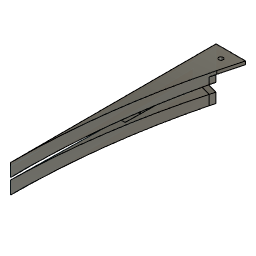
RampaZaKosuRavan v2 (Autodesk Fusion 360 design; units mm, degrees)
Autodesk Fusion 360 part; units mm, degrees
note: some values were not read from the file. Chosen so that the rebuilt part matches the saved one: which pieces of a blend or face edit are solid.
sketch "Sketch1" plane through (0, 0, 0) normal (0, 0, 1) x (1, 0, 0)
  line L0 (50, 20) -> (133, 20)
  line L1 (127.39759, 40.238898) -> (133, 20)
  line L2 (50, 20) -> (30, 20)
  line L3 (30, 20) -> (127.39759, 40.238898)
  dimension "d1" = 83
  dimension "d2" = 80
  dimension "d3" = 21
  constraint horizontal L0
  constraint parallel L0 L2
  measures "d1" distance of L0.start L0.end
extrude "Extrude1" add sketch "Sketch1" along normal blind 23 makes body 1
extrude "Extrude2" add 1 faces at (131.13253, 26.746299, 7.666667) along direction (0.96375706, 0.26678141, 0) blind 30 on bodies 1 bodies 1
sketch "Sketch2" plane through (157.589043, 43.622847, 0) normal (0.963757, 0.266781, 0) x (-0.266781, 0.963757, 0)
  line L0 (-16.206786, 0) -> (4.793214, 0)
  line L1 (4.793214, 0) -> (4.793214, 23)
  line L2 (4.793214, 23) -> (-16.206786, 23)
  line L3 (-16.206786, 23) -> (-16.206786, 0)
  line L4 (-16.206786, 23) -> (-16.206786, 20)
  line L5 (-16.206786, 20) -> (4.793214, 20)
  dimension "d8" = 3
  constraint perpendicular L2 L4
  constraint perpendicular L1 L5
extrude "Extrude3" cut sketch "Sketch2" against normal blind 30 contours L0 L1 L3 L5 picked at (-2.206786, 6.666667) bodies 1
sketch "Sketch3" plane through (0, 0, 23) normal (0, 0, 1) x (-1, 0, 0)
  line L0 (-30, -20) -> (-133, -20)
  line L1 (-133, -20) -> (-161.912712, -28.003442)
  line L2 (-161.912712, -28.003442) -> (-156.310302, -48.242341)
  line L3 (-156.310302, -48.242341) -> (-127.39759, -40.238898)
  line L4 (-127.39759, -40.238898) -> (-30, -20)
  line L5 (-156.310302, -48.242341) -> (-159.111507, -38.122892)
  line L6 (-159.111507, -38.122892) -> (-149.473936, -35.455077)
  circle A0 centre (-149.473936, -35.455077) radius 2
  dimension "d11" = 10.5
  dimension "d12" = 10
  dimension "d13" = 4
  constraint perpendicular L1 L5
  constraint perpendicular L2 L6
  measures "d13" diameter of A0
extrude "Extrude4" cut sketch "Sketch3" against normal blind 50 contours A0 picked at (-150.166062, -35.037269) bodies 1
sketch "Sketch4" plane through (0, 20, 0) normal (0, -1, 0) x (1, 0, 0)
  line L0 (30, 0) -> (133, 0)
  line L1 (133, 0) -> (133, 20)
  line L2 (133, 20) -> (133, 23)
  line L3 (133, 23) -> (30, 23)
  line L4 (30, 23) -> (30, 0)
  line L5 (133, 20) -> (133, 0)
  line L6 (133, 20) -> (133, 10)
  line L7 (133, 10) -> (30, 10)
  line L8 (30, 10) -> (30, 15)
  line L9 (30, 10) -> (30, 5)
  line L10 (30, 5) -> (133, 5)
  line L11 (133, 5) -> (30, 15)
  line L12 (30, 15) -> (133, 15)
  dimension "d16" = 10
  dimension "d17" = 5
  dimension "d18" = 5
  constraint coincident L1.end L2.start
  constraint coincident L0.end L1.start
  constraint perpendicular L0 L6
  constraint coincident L4 L7.end
  constraint perpendicular L4 L7
  constraint perpendicular L7 L8
  constraint perpendicular L7 L9
  constraint coincident L5 L10.end
  constraint perpendicular L5 L10
  constraint midpoint L6 L12.end
  measures "d16" distance of L1.end L6.end
  measures "d17" distance of L7.end L8.end
  measures "d18" distance of L7.end L9.end
extrude "Extrude5" cut sketch "Sketch4" against normal blind 8 contours L4 L7 L9 L10 L11 | L1 L5 L7 L11 | L4 L7 L8 L11 | L1 L5 L6 L7 L11 L12 picked at (81.5, 6.666667) picked at (115.833333, 8.333333) picked at (47.166667, 11.666667) picked at (81.5, 13.333333) bodies 1
sketch "Sketch5" plane through (0, 0, 0) normal (0, 0, -1) x (1, 0, 0)
  line L0 (127.39759, -40.238898) -> (133, -20)
  line L1 (133, -20) -> (30, -20)
  line L2 (30, -20) -> (127.39759, -40.238898)
  line L3 (30, -20) -> (0.627444, -13.89648)
  line L4 (0.627444, -13.89648) -> (81.5, -20)
  dimension "d21" = 30
  constraint coincident L1.end L2.start
  constraint parallel L2 L3
  constraint midpoint L1 L4.end
extrude "Extrude6" add sketch "Sketch5" against normal blind 2 contours L1 L3 L4 picked at (37.375815, -17.965493) bodies 1
extrude "Extrude7" add 1 faces at (37.375815, 17.965493, 2) along direction (0, 0, 1) blind 1 on bodies 1 bodies 1
sketch "Sketch6" plane through (0, 0, 23) normal (0, 0, 1) x (-1, 0, 0)
  circle A0 centre (-149.473936, -35.455077) radius 2
  line L0 (-30, -20) -> (-133, -20)
  line L1 (-133, -20) -> (-161.912712, -28.003442)
  line L2 (-161.912712, -28.003442) -> (-156.310302, -48.242341)
  line L3 (-156.310302, -48.242341) -> (-127.39759, -40.238898)
  line L4 (-127.39759, -40.238898) -> (-30, -20)
  line L5 (-30, -20) -> (-0.627444, -13.89648)
  line L6 (-0.627444, -13.89648) -> (-81.5, -20)
  dimension "d26" = 30
  constraint coincident L0.start L4.end
  constraint parallel L4 L5
  constraint midpoint L0 L6.end
extrude "Extrude8" add sketch "Sketch6" against normal blind 6 contours L0 L5 L6 picked at (-37.375815, -17.965493) bodies 1
sketch "Sketch7" plane through (0, 0, 0) normal (0, 0, -1) x (1, 0, 0)
  line L0 (127.39759, -40.238898) -> (133, -20)
  line L1 (133, -20) -> (81.5, -20)
  line L2 (81.5, -20) -> (0.627444, -13.89648)
  line L3 (0.627444, -13.89648) -> (127.39759, -40.238898)
  line L4 (0.627444, -13.89648) -> (-14.058834, -10.84472)
  line L5 (-14.058834, -10.84472) -> (41.063722, -16.94824)
  dimension "d30" = 15
  constraint parallel L3 L4
extrude "Extrude9" add sketch "Sketch7" against normal blind 2 contours L2 L4 L5 picked at (9.210777, -13.89648) bodies 1
sketch "Sketch8" plane through (0, 0, 23) normal (0, 0, 1) x (-1, 0, 0)
  circle A0 centre (-149.473936, -35.455077) radius 2
  line L0 (-81.5, -20) -> (-133, -20)
  line L1 (-133, -20) -> (-161.912712, -28.003442)
  line L2 (-161.912712, -28.003442) -> (-156.310302, -48.242341)
  line L3 (-156.310302, -48.242341) -> (-127.39759, -40.238898)
  line L4 (-127.39759, -40.238898) -> (-0.627444, -13.89648)
  line L5 (-0.627444, -13.89648) -> (-81.5, -20)
  line L6 (-0.627444, -13.89648) -> (14.058834, -10.84472)
  line L7 (-41.063722, -16.94824) -> (14.058834, -10.84472)
  dimension "d33" = 15
  constraint parallel L4 L6
extrude "Extrude10" add sketch "Sketch8" against normal blind 2 contours L5 L6 L7 picked at (-9.210777, -13.89648) bodies 1
sketch "Sketch9" plane through (0, 0, 0) normal (0, 0, 1) x (1, 0, 0)
  line L0 (0, 0) -> (27.195232, 0)
  line L1 (21.703887, -21) -> (0, -21)
  line L2 (0, -21) -> (0, 0)
  line L3 (0, -21) -> (0, -189.790785)
  line L4 (21.703887, -21) -> (27.195232, 0)
  line L5 (50, -50) -> (50, -133)
  line L6 (50, -50) -> (70.238898, -127.39759)
  line L7 (70.238898, -127.39759) -> (50, -133)
  line L8 (21.703887, -21) -> (0, -104) construction
  line L9 (20.238898, -26.60241) -> (0, -21) construction
  arc A0 (21.703887, -21) -> (0, -189.790785) centre (667.193566, -189.790785) ccw
  dimension "d37" = 83
  dimension "d38" = 80
  dimension "d39" = 21
  dimension "d40" = 83
  dimension "d41" = 21
  dimension "d42" = 80
  dimension "d43" = 21
  constraint coincident L0.start L2.end
  constraint horizontal L0
  constraint perpendicular L0 L2
  constraint perpendicular L1 L3
  constraint vertical L3
  constraint vertical L5
  constraint coincident L3 L8.end
  constraint collinear L4 L8
  constraint tangent L8 A0
  constraint tangent L3 A0
  measures "d37" distance of L5.start L5.end
  measures "d40" distance of L1 L8.end
  measures "d41" distance of L0 L1
extrude "Extrude11" add sketch "Sketch9" along normal blind 23 separate body contours L0 L1 L2 L4 | L1 L3 A0 picked at (16.299706, -7) picked at (10.45978, -39.525925) makes body 2
sketch "Sketch10" plane through (0, 0, 0) normal (-1, 0, 0) x (0, -1, 0)
  line L0 (0, 0) -> (189.790785, 0)
  line L1 (189.790785, 0) -> (189.790785, 23)
  line L2 (189.790785, 23) -> (0, 23)
  line L3 (0, 23) -> (0, 0)
  line L4 (189.790785, 0) -> (189.790785, 3)
  line L5 (189.790785, 3) -> (189.790785, 12)
  line L6 (189.790785, 12) -> (189.790785, 14)
  line L7 (189.790785, 14) -> (189.790785, 23)
  line L8 (0, 0) -> (21, 0)
  line L9 (21, 0) -> (21, 3)
  line L10 (21, 3) -> (21, 9)
  line L11 (21, 9) -> (21, 17)
  line L12 (21, 17) -> (21, 23)
  line L13 (21, 17) -> (189.790785, 14)
  line L14 (21, 9) -> (189.790785, 12)
  dimension "d46" = 3
  dimension "d47" = 9
  dimension "d48" = 2
  dimension "d49" = 21
  dimension "d50" = 3
  dimension "d51" = 6
  dimension "d52" = 8
  constraint perpendicular L0 L4
  constraint parallel L1 L5
  constraint parallel L1 L6
  constraint coincident L0.start L3.end
  constraint perpendicular L3 L8
  constraint perpendicular L8 L9
  constraint parallel L9 L10
  constraint parallel L10 L11
  constraint coincident L2 L12.end
  constraint perpendicular L2 L12
  measures "d49" distance of L0.start L8.end
  measures "d50" distance of L8.end L9.end
  measures "d51" distance of L9.end L10.end
  measures "d52" distance of L10.end L11.end
extrude "Extrude12" cut sketch "Sketch10" against normal blind 50 contours L1 L6 L11 L13 L14 picked at (77.263595, 13.333333) bodies 2
sketch "Sketch11" plane through (0, 0, 0) normal (-1, 0, 0) x (0, -1, 0)
  line L0 (21, 17) -> (189.790785, 14)
  line L1 (189.790785, 14) -> (189.790785, 23)
  line L2 (189.790785, 23) -> (0, 23)
  line L3 (0, 23) -> (0, 0)
  line L4 (0, 0) -> (189.790785, 0)
  line L5 (189.790785, 0) -> (189.790785, 12)
  line L6 (189.790785, 12) -> (21, 9)
  line L7 (21, 9) -> (21, 17)
extrude "Extrude13" cut 1 faces at (7.234629, -21, 11.666667) along direction (0, 1, 0) blind 50 on bodies 2 bodies 2
delete_face "DeleteFace1" 1 faces at (107.764783, 36.159266, 11.666667) on bodies 1
extrude "Extrude14" cut 1 faces at (21.703887, -7, 11.666667) along direction (1, 0, 0) blind 50 on bodies 2 bodies 2 makes body 3 at (10.45978, -32.525925, 23)
extrude "Extrude15" add 1 faces at (10.45978, -32.525925, 23) along direction (0, 0, 1) blind 3 on bodies 3 bodies 3
extrude "Extrude16" cut 1 faces at (16.299706, -7, 17) along direction (0, 0, 1) blind 6 on bodies 3 bodies 3
extrude "Extrude17" cut 1 faces at (16.299706, -7, 9) along direction (0, 0, -1) blind 6 on bodies 2 bodies 2
sketch "Sketch12" plane through (0, 0, 0) normal (0, 1, 0) x (1, 0, 0)
sketch "Sketch13" plane through (0, 0, 23) normal (0, 0, -1) x (1, 0, 0)
  line L0 (0, 0) -> (27.195232, 0)
  line L1 (27.195232, 0) -> (21.703887, 21)
  line L2 (21.703887, 21) -> (0, 21)
  line L3 (0, 21) -> (0, 0)
  line L4 (0, 21) -> (5.491345, 0)
  line L5 (0, 21) -> (21.703887, 21)
  line L6 (21.703887, 21) -> (10.903887, 21)
  line L7 (10.903887, 21) -> (0, 21)
  line L8 (10.903887, 21) -> (12.83906, 11.189031)
  circle A0 centre (12.83906, 11.189031) radius 2
  dimension "d65" = 10.8
  dimension "d66" = 10
  dimension "d67" = 4
  constraint coincident L2.end L3.start
  constraint parallel L1 L4
  constraint parallel L5 L6
  measures "d67" diameter of A0
extrude "Extrude18" cut sketch "Sketch13" against normal blind 50 contours A0 picked at (12.692597, 10.628692) bodies 3
sketch "Sketch14" plane through (0, 0, 26) normal (0, 0, 1) x (-1, 0, 0)
  circle A0 centre (-12.83906, 11.189031) radius 2
  line L0 (0, 0) -> (0, 189.790785)
  arc A1 (-21.703887, 21) -> (0, 189.790785) centre (-667.193566, 189.790785) ccw
  line L1 (-21.703887, 21) -> (-27.195232, 0)
  line L2 (-27.195232, 0) -> (0, 0)
  circle A2 centre (-12.83906, 11.189031) radius 2
  constraint concentric A0 A2
extrude "Extrude19" cut sketch "Sketch14" against normal blind 50 contours A0 A2 picked at (-12.266062, 10.716343) bodies 2
sketch "Sketch15" plane through (0, 0, 0) normal (0, 0, -1) x (1, 0, 0)
  circle A0 centre (12.83906, 11.189031) radius 2
  line L0 (0, 189.790785) -> (0, 0)
  line L1 (0, 0) -> (27.195232, 0)
  line L2 (27.195232, 0) -> (21.703887, 21)
  arc A1 (0, 189.790785) -> (21.703887, 21) centre (667.193566, 189.790785) ccw
  line L3 (0, 21) -> (0, 104)
  line L4 (0, 104) -> (20.26321, 26.608771)
  line L5 (20.26321, 26.608771) -> (0, 21)
  dimension "d72" = 83
  dimension "d73" = 80
  constraint coincident L0 L3.start
  measures "d72" distance of L3.start L3.end
extrude "Extrude20" cut sketch "Sketch15" against normal blind 23 contours L0 L1 L2 A1 L5 picked at (10.885743, 20.249219) bodies 2 3
sketch "Sketch16" plane through (0, 0, 23) normal (0, 0, -1) x (1, 0, 0)
  circle A0 centre (12.83906, 11.189031) radius 2
  line L0 (0, 0) -> (27.195232, 0)
  line L1 (27.195232, 0) -> (21.703887, 21)
  arc A1 (20.26321, 26.608771) -> (21.703887, 21) centre (667.193566, 189.790785) ccw
  line L2 (20.26321, 26.608771) -> (0, 21)
  line L3 (0, 21) -> (0, 0)
  circle A2 centre (12.83906, 11.189031) radius 2
  dimension "d76" = 4
  constraint concentric A0 A2
  measures "d76" diameter of A2
extrude "Extrude21" add sketch "Sketch16" against normal blind 3 contours A0 A2 picked at (13.412058, 10.716343) bodies 3
sketch "Sketch17" plane through (0, 0, 23) normal (0, 0, -1) x (1, 0, 0)
  line L0 (0, 0) -> (27.195232, 0)
  line L1 (27.195232, 0) -> (21.703887, 21)
  arc A0 (20.26321, 26.608771) -> (21.703887, 21) centre (667.193566, 189.790785) ccw
  line L2 (20.26321, 26.608771) -> (0, 21)
  line L3 (0, 21) -> (0, 0)
  line L4 (20.26321, 26.608771) -> (10.143714, 23.807737)
  line L5 (10.143714, 23.807737) -> (12.811365, 14.170122)
  circle A1 centre (12.811365, 14.170122) radius 2
  dimension "d79" = 10.5
  dimension "d80" = 10
  dimension "d81" = 4
  constraint parallel L2 L4
  constraint perpendicular L2 L5
  measures "d81" diameter of A1
extrude "Extrude22" cut sketch "Sketch17" against normal blind 50 contours A1 picked at (12.093403, 13.629509) bodies 3
sketch "Sketch18" plane through (-5.399058, -19.505564, 0) normal (0.266765, 0.963762, 0) x (-0.963762, 0.266765, 0)
  line L0 (-26.627196, 16.900313) -> (-5.602068, 17)
  line L1 (-5.602068, 17) -> (-5.602068, 23)
  line L2 (-5.602068, 23) -> (-26.627196, 23)
  line L3 (-26.627196, 23) -> (-26.627196, 16.900313)
  line L4 (-26.627196, 23) -> (-5.602068, 23)
  line L5 (-5.602068, 23) -> (-5.602068, 0)
  line L6 (-26.627196, 23) -> (-26.627196, 0)
  line L7 (-26.627196, 0) -> (-5.602068, 0)
  constraint perpendicular L4 L5
  constraint perpendicular L2 L6
  constraint perpendicular L5 L7
extrude "Extrude23" add sketch "Sketch18" along normal blind 5 bodies 2 3
sketch "Sketch19" plane through (0, 0, 23) normal (0, 0, -1) x (1, 0, 0)
  line L0 (21.504499, 21.764349) -> (1.333826, 16.181192)
  line L1 (1.333826, 16.181192) -> (0, 21)
  line L2 (0, 21) -> (0, 0)
  line L3 (0, 0) -> (27.195232, 0)
  line L4 (27.195232, 0) -> (21.703887, 21)
  arc A0 (21.504499, 21.764349) -> (21.703887, 21) centre (667.193566, 189.790785) ccw
  circle A1 centre (12.811365, 14.170122) radius 2
  circle A2 centre (12.811365, 14.170122) radius 2
  constraint concentric A1 A2
extrude "Extrude24" add sketch "Sketch19" against normal blind 3 contours A1 A2 picked at (13.384363, 13.697433) bodies 2
sketch "Sketch20" plane through (0, 0, 23) normal (0, 0, -1) x (1, 0, 0)
  line L0 (21.504499, 21.764349) -> (1.333826, 16.181192)
  line L1 (1.333826, 16.181192) -> (0, 21)
  line L2 (0, 21) -> (0, 0)
  line L3 (0, 0) -> (27.195232, 0)
  line L4 (27.195232, 0) -> (21.703887, 21)
  arc A0 (21.504499, 21.764349) -> (21.703887, 21) centre (667.193566, 189.790785) ccw
  line L5 (21.504499, 21.764349) -> (11.346065, 19.107994)
  line L6 (11.346065, 19.107994) -> (14.013716, 9.470378)
  circle A1 centre (14.013716, 9.470378) radius 2
  dimension "d88" = 10.5
  dimension "d89" = 10
  dimension "d90" = 4
  constraint perpendicular L4 L5
  constraint perpendicular L0 L6
  measures "d90" diameter of A1
extrude "Extrude25" cut sketch "Sketch20" against normal blind 50 contours A1 picked at (12.632766, 9.80047) bodies 2
sketch "Sketch21" plane through (25.662268, -7.103208, 0) normal (0.963762, -0.266765, 0) x (0.266765, 0.963762, 0)
  line L0 (-20.238993, 23) -> (-20.238993, 16.900313)
  line L1 (-20.238993, 16.900313) -> (-20.238993, 9.099687)
  line L2 (-20.238993, 9.099687) -> (-20.238993, 0)
  line L3 (-20.238993, 0) -> (-15.238993, 0)
  line L4 (-15.238993, 0) -> (-15.238993, 23)
  line L5 (-15.238993, 23) -> (-20.238993, 23)
  line L6 (-20.238993, 16.900313) -> (-15.238993, 16.900313)
  line L7 (-20.238993, 9.099687) -> (-15.238993, 9.099687)
  constraint perpendicular L4 L6
  constraint perpendicular L4 L7
extrude "Extrude26" cut sketch "Sketch21" against normal blind 10 contours L1 L4 L6 L7 picked at (-18.572326, 11.699896) bodies 2
sketch "Sketch22" plane through (0, 0, 0) normal (-1, 0, 0) x (0, -1, 0)
  line L0 (21, 9) -> (89.024246, 10.204617)
  line L1 (89.024246, 10.204617) -> (88.925534, 15.778848)
  line L2 (88.925534, 15.778848) -> (21, 17)
  line L3 (21, 17) -> (21, 9)
  constraint perpendicular L0 L1
  constraint vertical L3
extrude "Extrude27" cut sketch "Sketch22" against normal blind 5 bodies 2
sketch "Sketch23" plane through (0, 0, 0) normal (-1, 0, 0) x (0, -1, 0)
  line L0 (21, 9) -> (21, 17)
  line L1 (21, 17) -> (75.000001, 16)
  line L2 (75.000001, 16) -> (74.888312, 9.968796)
  line L3 (74.888312, 9.968796) -> (21, 9)
  constraint vertical L0
  constraint perpendicular L1 L2
extrude "Extrude28" add sketch "Sketch23" against normal blind 5 bodies 2
hidden bodies 1
